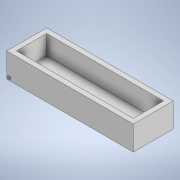
# Autodesk Inventor part: GiveBox
Saved by Autodesk Inventor 2021 (Build 250183000, 183)
## iProperties
Created: 2020-08-04
Part Number: GiveBox
Material: Generic
Document SubType Name: Modeling
Designer: karim
Density: 1 g/cm^3
Appearance: Default
Author: karim
Autodesk Inventor part; units mm, degrees
ref_plane "YZ Plane" through (0, 0, 0) normal (1, 0, 0) x (0, 1, 0)
ref_plane "XZ Plane" through (0, 0, 0) normal (0, 1, 0) x (-1, 0, 0)
ref_plane "XY Plane" through (0, 0, 0) normal (0, 0, 1) x (1, 0, 0)
sketch "Sketch1" plane through (0, 0, 0) normal (0, 1, 0) x (-1, 0, 0)
  line L0 (120, 31) -> (-120, 31)
  line L1 (-120, 31) -> (-120, -31)
  line L2 (-120, -31) -> (120, -31)
  line L3 (120, -31) -> (120, 31)
  line L4 (120, 31) -> (-120, -31) construction
  line L5 (-120, 31) -> (120, -31) construction
  line L6 (130, 41) -> (-130, 41)
  line L7 (-130, 41) -> (-130, -41)
  line L8 (-130, -41) -> (130, -41)
  line L9 (130, -41) -> (130, 41)
  point P0 (0, 0)
  dimension "d0" = 62
  dimension "d1" = 240
  dimension "d2" = 10
  constraints: 20 end point, 4 parallel, 2 midpoint, 2 perpendicular, 1 horizontal, 3 other
  measures "d0" distance of L0.end L1.end
  measures "d1" distance of L1.end L2.end
  measures "d2" distance between parallel lines of L3 L9
extrude "Extrusion1" add sketch "Sketch1" along normal blind 10 contours L3 L2 L1 L0
extrude "Extrusion2" add sketch "Sketch1" along normal blind 50
sketch "Sketch2" plane through (-130, 0, 41) normal (0, 0, 1) x (1, 0, 0)
  circle A0 centre (5, 5) radius 3.2
  line L0 (0, 0) -> (0, 50) projected
  line L1 (0, 0) -> (260, 0) projected
  point P0 (130, 0)
  dimension "d9" = 6.4
  dimension "d22" = 5
  dimension "d23" = 5
  constraints: 1 centre point
  measures "d9" diameter of A0
  measures "d22" distance from line of L0 A0.centre
  measures "d23" distance from line of L1 A0.centre
extrude "Extrusion3" cut sketch "Sketch2" against normal through all
sketch "Sketch3" plane through (0, 0, 0) normal (0, -1, 0) x (1, 0, 0)
  point P0 (0, 0)
body "Solid1"
